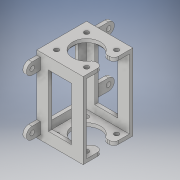
# Autodesk Inventor part: 14HM11 Chassis
Saved by Autodesk Inventor 2019 (Build 230136000, 136)
## iProperties
Created: 2018-11-12
Part Number: 14HM11 Chassis
Material: Generic
Document SubType Name: Modeling
Designer: Billy
Density: 1 g/cm^3
Appearance: Default
Author: Billy
Autodesk Inventor part; units mm, degrees
ref_plane "YZ Plane" through (0, 0, 0) normal (1, 0, 0) x (0, 1, 0)
ref_plane "XZ Plane" through (0, 0, 0) normal (0, 1, 0) x (-1, 0, 0)
ref_plane "XY Plane" through (0, 0, 0) normal (0, 0, 1) x (1, 0, 0)
sketch "Sketch1" plane through (0, 0, 0) normal (0, 1, 0) x (-1, 0, 0)
  line L0 (0, 0) -> (-37, 0)
  line L1 (-37, 0) -> (-37, -37)
  line L2 (-37, -37) -> (0, -37)
  line L3 (0, -37) -> (0, 0)
  circle A0 centre (-5.5, -5.5) radius 2
  circle A1 centre (-5.5, -31.5) radius 2
  circle A2 centre (-31.5, -5.5) radius 2
  circle A3 centre (-31.5, -31.5) radius 2
  circle A4 centre (-18.5, -18.5) radius 12
  dimension "d10" = 24
  constraints: 8 end point, 5 centre point, 2 parallel, 1 horizontal, 1 perpendicular
  measures "d10" diameter of A4
extrude "Extrusion1" add sketch "Sketch1" along normal blind 3
sketch "Sketch2" plane through (0, 3, 0) normal (0, 1, 0) x (1, 0, 0)
  circle A0 centre (18.5, 18.5) radius 12
  circle A1 centre (31.5, 31.5) radius 2
  circle A2 centre (31.5, 5.5) radius 2
  circle A3 centre (5.5, 31.5) radius 2
  circle A4 centre (5.5, 5.5) radius 2
  line L0 (0, 0) -> (37, 0)
  line L1 (37, 37) -> (0, 37)
  line L2 (0, 37) -> (0, 0)
  line L3 (-3, -3) -> (37, -3)
  line L4 (37, 40) -> (-3, 40)
  line L5 (-3, 40) -> (-3, -3)
  line L6 (37, -3) -> (37, 0)
  line L7 (37, 37) -> (37, 40)
  dimension "d13" = 3
  constraints: 16 end point, 9 centre point
  measures "d13" distance between parallel lines of L2 L5
extrude "Extrusion2" add sketch "Sketch2" along normal blind 60 and the other way blind 3 contours L0 L6 L3 L5 L4 L7 L1 L2
sketch "Sketch4" plane through (0, 63, 0) normal (0, 1, 0) x (1, 0, 0)
  circle A0 centre (18.5, 18.5) radius 12 projected
  circle A1 centre (31.5, 31.5) radius 2 projected
  circle A2 centre (31.5, 5.5) radius 2 projected
  circle A3 centre (5.5, 31.5) radius 2 projected
  circle A4 centre (5.5, 5.5) radius 2 projected
  line L0 (0, 0) -> (37, 0) projected
  line L1 (37, 0) -> (37, 37) projected
  line L2 (37, 37) -> (0, 37) projected
  line L3 (0, 37) -> (0, 0) projected
  line L4 (37, 0) -> (0, 0) projected
  line L5 (0, 0) -> (0, 37) projected
  line L6 (0, 37) -> (37, 37) projected
  line L7 (37, 37) -> (37, 40) projected
  line L8 (37, 40) -> (-3, 40) projected
  line L9 (-3, 40) -> (-3, -3) projected
  line L10 (-3, -3) -> (37, -3) projected
  line L11 (37, -3) -> (37, 0) projected
extrude "Extrusion3" add sketch "Sketch4" along normal blind 3
sketch "Sketch5" plane through (0, 66, 0) normal (0, 1, 0) x (1, 0, 0)
  arc A0 (29.4087, 13.5) -> (29.4087, 23.5) centre (18.5, 18.5) ccw
  circle A1 centre (5.5, 5.5) radius 2
  circle A2 centre (5.5, 31.5) radius 2
  circle A3 centre (31.5, 5.5) radius 2
  circle A4 centre (31.5, 31.5) radius 2
  line L0 (37, 13.5) -> (37, 23.5)
  line L1 (37, 40) -> (-3, 40)
  line L2 (-3, 40) -> (-3, -3)
  line L3 (-3, -3) -> (37, -3)
  arc A5 (29.4087, 13.5) -> (29.4087, 23.5) centre (18.5, 18.5) ccw
  line L4 (37, 23.5) -> (37, 13.5)
  line L5 (29.4087, 23.5) -> (37, 23.5)
  line L6 (29.4087, 13.5) -> (37, 13.5)
  point P0 (0, 0)
  constraints: 14 end point, 10 centre point, 4 point on circle
extrude "Extrusion4" cut sketch "Sketch5" against normal up to surface (66 mm away) contours A0 L5 L0 L6
fillet "Fillet1" radius 4 8 edges at (29.4087, 64.5, -13.5) (37, 64.5, -13.5) (37, 64.5, -23.5) (29.4087, 64.5, -23.5) (37, 1.5, -13.5) (29.4087, 1.5, -13.5) (37, 1.5, -23.5) (29.4087, 1.5, -23.5)
sketch "Sketch7" plane through (37, 0, -40) normal (0, 0, -1) x (-1, 0, 0)
  line L0 (40, 66) -> (40, 0) projected
  line L1 (0, 66) -> (40, 66) projected
  line L2 (0, 66) -> (0, 0) projected
  line L3 (40, 0) -> (0, 0) projected
  line L4 (30, 56) -> (30, 10)
  line L5 (30, 10) -> (10, 10)
  line L6 (10, 10) -> (10, 56)
  line L7 (10, 56) -> (30, 56)
  point P0 (37, 0)
  dimension "d26" = 10
  constraints: 8 end point, 3 other
  measures "d26" distance between parallel lines of L1 L7
extrude "Extrusion5" cut sketch "Sketch7" against normal up to surface (43 mm away) contours L4 L5 L6 L7
sketch "Sketch8" plane through (-3, 0, -40) normal (-1, 0, 0) x (0, 0, 1)
  line L0 (43, 66) -> (43, 0) projected
  line L1 (0, 66) -> (43, 66) projected
  line L2 (0, 66) -> (0, 0) projected
  line L3 (43, 0) -> (0, 0) projected
  line L4 (33, 56) -> (33, 10)
  line L5 (33, 10) -> (10, 10)
  line L6 (10, 10) -> (10, 56)
  line L7 (10, 56) -> (33, 56)
  point P0 (40, 0)
  dimension "d29" = 10
  constraints: 8 end point, 3 other
  measures "d29" distance between parallel lines of L1 L7
extrude "Extrusion6" cut sketch "Sketch8" against normal blind 3 contours L4 L5 L6 L7
sketch "Sketch9" plane through (-3, 0, -40) normal (-1, 0, 0) x (0, 0, 1)
  line L0 (10, 56) -> (33, 56)
  line L1 (33, 56) -> (33, 10)
  line L2 (33, 10) -> (10, 10)
  line L3 (10, 10) -> (10, 56)
  line L4 (0, 66) -> (43, 66)
  line L5 (43, 0) -> (0, 0)
  line L6 (0, 66) -> (43, 66) projected
  circle A0 centre (50.075, 8.87) radius 2
  circle A1 centre (-15.965, 12.045) radius 2
  circle A2 centre (50.075, 57.13) radius 2
  circle A3 centre (-15.965, 53.955) radius 2
  arc A4 (50.075, 3.87) -> (50.075, 13.87) centre (50.075, 8.87) ccw
  arc A5 (50.075, 52.13) -> (50.075, 62.13) centre (50.075, 57.13) ccw
  arc A6 (-15.965, 17.045) -> (-15.965, 7.045) centre (-15.965, 12.045) ccw
  arc A7 (-15.965, 58.955) -> (-15.965, 48.955) centre (-15.965, 53.955) ccw
  line L7 (50.075, 3.87) -> (43, 3.87)
  line L8 (50.075, 13.87) -> (43, 13.87)
  line L9 (50.075, 62.13) -> (43, 62.13)
  line L10 (50.075, 52.13) -> (43, 52.13)
  line L11 (-15.965, 7.045) -> (0, 7.045)
  line L12 (-15.965, 17.045) -> (0, 17.045)
  line L13 (-15.965, 48.955) -> (0, 48.955)
  line L14 (0, 56) -> (0, 10) projected
  line L15 (-15.965, 58.955) -> (0, 58.955)
  line L16 (0, 66) -> (0, 0) projected
  line L17 (0, 58.955) -> (0, 48.955)
  line L18 (0, 17.045) -> (0, 7.045)
  line L19 (43, 62.13) -> (43, 52.13)
  line L20 (43, 13.87) -> (43, 3.87)
  point P0 (40, 0)
  dimension "d53" = 10
  constraints: 36 end point, 9 coincident, 8 centre point, 8 perpendicular, 8 point on circle, 4 tangent, 3 parallel, 2 point on line, 1 horizontal
  measures "d53" diameter of A6
extrude "Extrusion7" add sketch "Sketch9" against normal blind 3 contours L7 L20 L8 A4 | L10 L19 L9 A5 | L12 L14 L16 L11 A6 | L13 A7 L15 L16 L14
body "Solid1"
